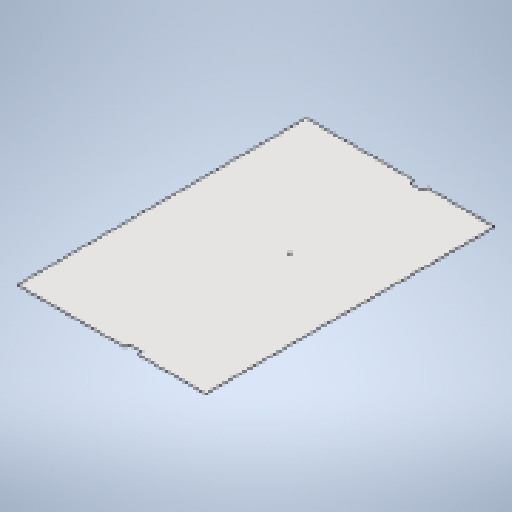
# Autodesk Inventor part: GnG frame 2 floor sheet 9
Saved by Autodesk Inventor 2025 (Build 290162010, 162A)
## iProperties
Created: 2025-10-28
Part Number: GnG frame 2 floor sheet 9
Material: Stainless Steel
Document SubType Name: Sheet Metal
Designer: admin
Mass: 280.619 g
Surface Area: 364.406 cm^2
Volume: 35.0774 cm^3
Density: 8 g/cm^3
Sheet Metal Rule: AISI304 3mm Die 32
Sheet Metal Width: 1500,000 mm
Sheet Metal Length: 2300,000 mm
Sheet Metal Area: 3450000,000 mm^2
Appearance: Default
Flat Pattern Width: 150 cm
Flat Pattern Length: 230 cm
Flat Pattern Area: 34500 cm^2
Author: admin
Autodesk Inventor part; units mm, degrees
ref_plane "YZ Plane" through (0, 0, 0) normal (1, 0, 0) x (0, 1, 0)
ref_plane "XZ Plane" through (0, 0, 0) normal (0, 1, 0) x (-1, 0, 0)
ref_plane "XY Plane" through (0, 0, 0) normal (0, 0, 1) x (1, 0, 0)
sketch "Sketch1" plane through (0, 0, 0) normal (0, 0, 1) x (1, 0, 0)
  line L0 (0, 0) -> (-1500, 0)
  line L1 (-1500, 0) -> (-1500, -2300)
  line L2 (-1500, -2300) -> (0, -2300)
  line L3 (0, -2300) -> (0, 0)
  line L4 (0, 0) -> (-40, 0)
  line L5 (-40, 0) -> (-40, -35)
  line L6 (-40, -35) -> (0, -35)
  line L7 (0, -35) -> (0, 0)
  line L8 (0, -2300) -> (-40, -2300)
  line L9 (-40, -2300) -> (-40, -2265)
  line L10 (-40, -2265) -> (0, -2265)
  line L11 (0, -2265) -> (0, -2300)
  line L12 (-1500, 0) -> (-1460, 0)
  line L13 (-1460, 0) -> (-1460, -35)
  line L14 (-1460, -35) -> (-1500, -35)
  line L15 (-1500, -35) -> (-1500, 0)
  line L16 (-1500, -2300) -> (-1460, -2300)
  line L17 (-1460, -2300) -> (-1460, -2265)
  line L18 (-1460, -2265) -> (-1500, -2265)
  line L19 (-1500, -2265) -> (-1500, -2300)
  line L20 (-640, -2300) -> (-540, -2300)
  line L21 (-540, -2300) -> (-540, -2265)
  line L22 (-540, -2265) -> (-640, -2265)
  line L23 (-640, -2265) -> (-640, -2300)
  line L24 (-640, 0) -> (-540, 0)
  line L25 (-540, 0) -> (-540, -35)
  line L26 (-540, -35) -> (-640, -35)
  line L27 (-640, -35) -> (-640, 0)
  point P0 (0, -35)
  point P1 (-40, 0)
  point P2 (-40, -2300)
  point P3 (0, -2265)
  point P4 (-540, -2300)
  point P5 (-540, 0)
  point P6 (-1460, 0)
  point P7 (-1500, -35)
  dimension "d22" = 1500
  dimension "d23" = 2300
  dimension "d24" = 40
  dimension "d25" = 35
  dimension "d28" = 100
  dimension "d29" = 500
  measures "d22" distance of L2.end L1.end
  measures "d23" distance of L1.end L0.end
  measures "d24" distance of L6.end L5.end
  measures "d25" distance of L5.end L4.end
  measures "d28" distance of L25.end L26.end
  measures "d29" distance between parallel lines of L5 L25
extrude "Plate1" add sketch "Sketch1" along normal blind 3 contours L3 L6 L5 L0 | L5 L6 L3 L10 L9 L2 L21 L22 L23 L17 L18 L1 L14 L13 L0 L27 L26 L25 | L3 L2 L9 L10 | L13 L14 L1 L0 | L18 L17 L2 L1
sketch "Sketch5" plane through (0, 0, 3) normal (0, 0, 1) x (1, 0, 0)
  line L0 (0, 0) -> (-100, 0) construction
  line L1 (-100, 0) -> (-100, -5) construction
  line L2 (-100, -5) -> (0, -5) construction
  line L3 (0, -5) -> (0, 0) construction
  line L4 (-100, 0) -> (-101.3084, -4.1277)
  arc A0 (-103.6916, -4.1277) -> (-101.3084, -4.1277) centre (-102.5, -3.75) ccw
  line L5 (-103.6916, -4.1277) -> (-105, 0)
  line L6 (-105, 0) -> (-100, 0)
  line L7 (-105, 0) -> (-110, 0) construction
  line L8 (-110, 0) -> (-115, 0)
  line L9 (-115, 0) -> (-115, -5)
  line L10 (-115, -5) -> (-110, -5)
  line L11 (-110, -5) -> (-110, 0)
  line L12 (-115, 0) -> (-120, 0) construction
  line L13 (-120, 0) -> (-125, 0)
  line L14 (-125, 0) -> (-125, -5)
  line L15 (-125, -5) -> (-120, -5)
  line L16 (-120, -5) -> (-120, 0)
  line L17 (-125, 0) -> (-130, 0) construction
  line L18 (-130, 0) -> (-135, 0)
  line L19 (-135, 0) -> (-135, -5)
  line L20 (-135, -5) -> (-130, -5)
  line L21 (-130, -5) -> (-130, 0)
  line L22 (-135, 0) -> (-140, 0) construction
  line L23 (-140, 0) -> (-145, 0)
  line L24 (-145, 0) -> (-145, -5)
  line L25 (-145, -5) -> (-140, -5)
  line L26 (-140, -5) -> (-140, 0)
  line L27 (-145, 0) -> (-150, 0) construction
  line L28 (-150, 0) -> (-155, 0) construction
  circle A1 centre (-150, 0) radius 2.5
  point P0 (-102.5, 0)
  dimension "d30" = 100
  dimension "d31" = 5
  dimension "d32" = 5
  dimension "d33" = 5
  dimension "d34" = 1.25
  dimension "d35" = 5
  dimension "d36" = 5
  dimension "d37" = 5
  dimension "d38" = 5
  constraints: 58 end point, 11 horizontal, 10 equal length, 10 parallel, 5 perpendicular, 3 coincident, 3 tangent, 2 centre point, 2 point on circle, 1 midpoint, 1 point on line, 1 vertical alignment
  measures "d30" distance of L2.end L1.end
  measures "d31" distance of L1.end L0.end
  measures "d32" distance of L9.end L9.start
  measures "d33" distance of L5.end L0.end
  measures "d34" radius of A0
  measures "d35" distance of L15.start L13.end
  measures "d36" distance of L19.end L19.start
  measures "d37" distance of L24.end L24.start
  measures "d38" diameter of A1
extrude "Cut1" cut sketch "Sketch5" against normal blind 3 contours L4 A0 L5 L6 | L11 L10 L9 L8 | A1
sketch "Sketch6" plane through (0, 0, 3) normal (0, 0, 1) x (1, 0, 0)
  arc A0 (-152.5, 0) -> (-147.5, 0) centre (-150, 0) ccw construction
  line L0 (-540, 0) -> (-152.5, 0) construction
  line L1 (-1500, -2300) -> (-1500, 0) construction
  line L2 (0, -2300) -> (-540, -2300) construction
  line L3 (0, 0) -> (0, -2300) construction
  line L4 (-100, 0) -> (0, 0) construction
  line L5 (-100, 0) -> (-101.3084, -4.1277) construction
  arc A1 (-103.6916, -4.1277) -> (-101.3084, -4.1277) centre (-102.5, -3.75) ccw construction
  line L6 (-103.6916, -4.1277) -> (-105, 0) construction
  line L7 (-110, 0) -> (-105, 0) construction
  line L8 (-110, 0) -> (-110, -5) construction
  line L9 (-110, -5) -> (-115, -5) construction
  line L10 (-115, -5) -> (-115, 0) construction
  line L11 (-147.5, 0) -> (-115, 0) construction
  circle A2 centre (-520, -2100) radius 7.5
  line L12 (-540, -35) -> (-540, 0) construction
  line L13 (-640, -35) -> (-540, -35) construction
  line L14 (-640, 0) -> (-640, -35) construction
  line L15 (-1500, 0) -> (-640, 0) construction
  line L16 (-640, -2300) -> (-1500, -2300) construction
  line L17 (-640, -2265) -> (-640, -2300) construction
  line L18 (-540, -2265) -> (-640, -2265) construction
  line L19 (-540, -2300) -> (-540, -2265) construction
  line L20 (-520, -2300) -> (-520, 0) construction
  line L21 (-1070, 0) -> (-1070, -2300) construction
  line L22 (-1500, -1675) -> (0, -1675) construction
  line L23 (-1500, -1000) -> (0, -1000) construction
  circle A3 centre (-1070, -2100) radius 7.5
  circle A4 centre (-1300, -1675) radius 7.5
  circle A5 centre (-1300, -1000) radius 7.5
  circle A6 centre (-520, -1900) radius 7.5
  circle A7 centre (-1070, -1900) radius 7.5
  circle A8 centre (-520, -1700) radius 7.5
  circle A9 centre (-1070, -1700) radius 7.5
  circle A10 centre (-520, -1500) radius 7.5
  circle A11 centre (-1070, -1500) radius 7.5
  circle A12 centre (-520, -1300) radius 7.5
  circle A13 centre (-1070, -1300) radius 7.5
  circle A14 centre (-520, -1100) radius 7.5
  circle A15 centre (-1070, -1100) radius 7.5
  circle A16 centre (-520, -900) radius 7.5
  circle A17 centre (-1070, -900) radius 7.5
  circle A18 centre (-520, -700) radius 7.5
  circle A19 centre (-1070, -700) radius 7.5
  circle A20 centre (-520, -500) radius 7.5
  circle A21 centre (-1070, -500) radius 7.5
  circle A22 centre (-520, -300) radius 7.5
  circle A23 centre (-1070, -300) radius 7.5
  circle A24 centre (-520, -100) radius 7.5
  circle A25 centre (-1070, -100) radius 7.5
  circle A26 centre (-1100, -1675) radius 7.5
  circle A27 centre (-1100, -1000) radius 7.5
  circle A28 centre (-900, -1675) radius 7.5
  circle A29 centre (-900, -1000) radius 7.5
  circle A30 centre (-700, -1675) radius 7.5
  circle A31 centre (-700, -1000) radius 7.5
  circle A32 centre (-500, -1675) radius 7.5
  circle A33 centre (-500, -1000) radius 7.5
  circle A34 centre (-300, -1675) radius 7.5
  circle A35 centre (-300, -1000) radius 7.5
  circle A36 centre (-100, -1675) radius 7.5
  circle A37 centre (-100, -1000) radius 7.5
  dimension "d41" = 15
  dimension "d46" = 520
  dimension "d47" = 1070
  dimension "d48" = 625
  dimension "d49" = 1300
  dimension "d50" = 200
  dimension "d51" = 200
  dimension "d54" = 200
  dimension "d61" = 200
  constraints: 36 centre point, 10 point on line, 8 end point, 4 perpendicular, 3 equal radius, 2 midpoint, 1 horizontal, 1 horizontal alignment, 1 vertical, 1 vertical alignment, 64 other
  measures "d41" diameter of A2
  measures "d46" distance between parallel lines of L20 L3
  measures "d47" distance between parallel lines of L21 L3
  measures "d48" distance between parallel lines of L16 L22
  measures "d49" distance between parallel lines of L23 L16
  measures "d50" distance from line of L2 A2.centre
  measures "d51" distance from line of L1 A4.centre
  measures "d54" distance of A2.centre A6.centre
  measures "d61" distance of A4.centre A26.centre
extrude "Cut2" cut sketch "Sketch6" against normal blind 3 contours A3 | A4 | A5 | A6 | A7 | A8 | A9 | A10 | A11 | A12 | A13 | A14 | A15 | A16 | A17 | A18 | A19 | A20 | A21 | A22 | A23 | A24 | A25 | A26 | A27 | A28 | A29 | A30 | A31 | A32 | A33 | A34 | A35 | A36 | A37
equation "\"d34\" = 0.25 * d31"
equation "\"d39\" = Thickness"
equation "\"d54\" = d50"
equation "\"d61\" = d54"
equation "\"d44\" = Thickness"
equation "\"d2\" = Thickness"
equation "\"BendReliefWidth\" = Thickness"
equation "\"BendReliefDepth\" = 0.5 * Thickness"
equation "\"CornerReliefSize\" = 4 * Thickness"
equation "\"MinimumRemnant\" = 2 * Thickness"
equation "\"TransitionRadius\" = BendRadius"
equation "\"JacobiRadiusSize\" = BendRadius"
equation "\"GapSize\" = Thickness"
equation "\"Thickness\" = 3"
equation "\"BendRadius\" = 5"
body "Solid1"
